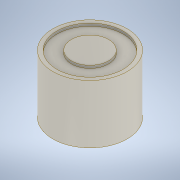
# Autodesk Inventor part: магнит
Saved by Autodesk Inventor 2020.1 (Build 241239000, 239)
## iProperties
Created: 2021-08-17
Part Number: магнит
Material: Титан
Document SubType Name: Modeling
Designer: Ni3na
Density: 4.51 g/cm^3
Appearance: Титан
Author: Ni3na
Autodesk Inventor part; units mm, degrees
ref_plane "YZ Plane" through (0, 0, 0) normal (1, 0, 0) x (0, 1, 0)
ref_plane "XZ Plane" through (0, 0, 0) normal (0, 1, 0) x (-1, 0, 0)
ref_plane "XY Plane" through (0, 0, 0) normal (0, 0, 1) x (1, 0, 0)
sketch "Эскиз1" plane through (0, 0, 0) normal (0, 1, 0) x (-1, 0, 0)
  circle A0 centre (7.4029, -9.7102) radius 14
  point P0 (0, 0)
  dimension "d0" = 28
  constraints: 1 centre point
  measures "d0" diameter of A0
extrude "Выдавливание1" add sketch "Эскиз1" along normal blind 22
sketch "Эскиз2" plane through (-7.4029, 22, -9.7102) normal (0, 1, 0) x (1, 0, 0)
  circle A0 centre (0, 0) radius 12.5
  circle A1 centre (0, 0) radius 7
  point P0 (7.4029, -9.7102)
  dimension "d6" = 25
  dimension "d7" = 14
  constraints: 2 centre point, 1 coincident
  measures "d6" diameter of A0
  measures "d7" diameter of A1
extrude "Выдавливание2" cut sketch "Эскиз2" against normal blind 1
sketch "Эскиз3" plane through (-7.4029, 0, -9.7102) normal (0, -1, 0) x (1, 0, 0)
  circle A0 centre (0, 0) radius 4
  circle A1 centre (0, 0) radius 3.5
  point P0 (7.4029, 9.7102)
  dimension "d8" = 8
  dimension "d9" = 7
  constraints: 2 centre point, 1 coincident
  measures "d8" diameter of A0
  measures "d9" diameter of A1
extrude "Выдавливание3" add sketch "Эскиз3" along normal blind 4
